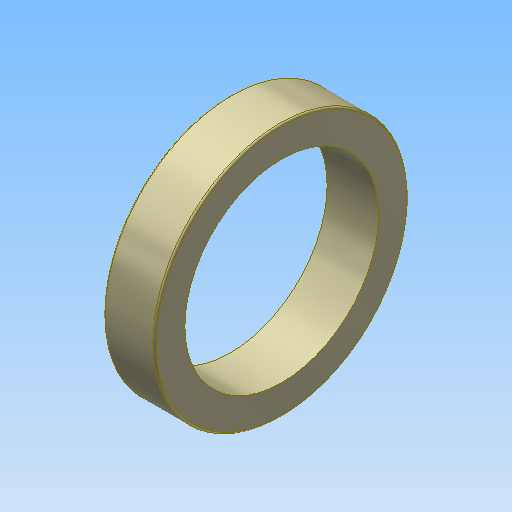
# Autodesk Inventor part: Collar_Seal_Inner
Saved by Autodesk Inventor 2020.1 (Build 241239000, 239)
## iProperties
Created: 2001-02-20
Part Number: Collar_Seal_Inner
Material: Nylon-6/6
Document SubType Name: Modeling
Designer: Joe M
Description: Piston rod packing
Engineer: Joe M
Density: 1.13 g/cm^3
Appearance: Nylon 6
Control State: 0
Master: False
Checked Out: False
Shininess: 31.0
Length Units: 11269
Angle Units: 11279
Time Units: 11290
Mass Units: 11283
Length Display Precision: 3
Angle Display Precision: 2
Compacted: True
Density: 1.13
Volumn: 4.935073823646865
Area: 31.043917378897465
PropertySet Name: Model Information
Title: Kolvstångstätning
Author: Joe M
Autodesk Inventor part; units mm, degrees
ref_plane "YZ Plane" through (0, 0, 0) normal (1, 0, 0) x (0, 1, 0)
ref_plane "XZ Plane" through (0, 0, 0) normal (0, 1, 0) x (-1, 0, 0)
ref_plane "XY Plane" through (0, 0, 0) normal (0, 0, 1) x (1, 0, 0)
sketch "Sketch1" plane through (0, 0, 0) normal (0, 0, 1) x (1, 0, 0)
  line L0 (0, 16) -> (8.5, 16)
  line L1 (8.5, 16) -> (8.5, 21)
  line L2 (8.5, 21) -> (0, 21)
  line L3 (0, 21) -> (0, 16)
  line L4 (0, 0) -> (32.3907, 0)
  dimension "d0" = 32
  dimension "d1" = 42
  dimension "d2" = 8.5
  constraints: 10 end point, 2 parallel, 2 perpendicular, 1 coincident, 1 horizontal, 1 vertical alignment
  measures "d0" diameter of L0 L4
  measures "d1" diameter of L2 L4
  measures "d2" distance of L1.end L2.end
revolve "Revolution1" add sketch "Sketch1" angle 360 about axis through (0, 0, 0) along (1, 0, 0)
fillet "Fillet1" radius 0.3 2 edges at (8.5, -21, 0) (0, -21, 0)
body "Solid1"
